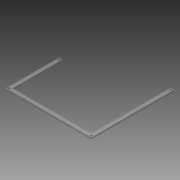
# Autodesk Inventor part: Bottom Plate
Saved by Autodesk Inventor 2013 (Build 170138000, 138)
## iProperties
Created: 2013-01-27
Part Number: Bottom Plate
Material: Polycarbonate, Clear
Document SubType Name: Modeling
Designer: Andrew Toennies
Density: 1.2 g/cm^3
Mass: 75.8926 g
Surface Area: 308.467 cm^2
Volume: 63.2438 cm^3
Author: Andrew Toennies
Autodesk Inventor part; units mm, degrees
ref_plane "YZ Plane" through (0, 0, 0) normal (1, 0, 0) x (0, 1, 0)
ref_plane "XZ Plane" through (0, 0, 0) normal (0, 1, 0) x (-1, 0, 0)
ref_plane "XY Plane" through (0, 0, 0) normal (0, 0, 1) x (1, 0, 0)
sketch "Sketch1" plane through (0, 0, 0) normal (0, 1, 0) x (-1, 0, 0)
  circle A0 centre (0, 0) radius 139.7
  line L0 (-146.05, 146.05) -> (-146.05, -146.05)
  line L1 (-146.05, -146.05) -> (0, -146.05)
  line L2 (-158.75, 158.75) -> (-158.75, -158.75)
  line L3 (-158.75, -158.75) -> (0, -158.75)
  line L4 (0, -158.75) -> (0, -146.05)
  line L5 (-146.05, 146.05) -> (146.05, 146.05)
  line L6 (146.05, 146.05) -> (146.05, -38.1)
  line L7 (146.05, -38.1) -> (158.75, -38.1)
  line L8 (158.75, -38.1) -> (158.75, 158.75)
  line L9 (158.75, 158.75) -> (-158.75, 158.75)
  dimension "d0" = 279.4
  dimension "d2" = 146.05
  dimension "d4" = 146.05
  dimension "d6" = 0
  dimension "d9" = 317.5
  dimension "d30" = 12.7
  dimension "d31" = 292.1
  dimension "d32" = 184.15
  dimension "d33" = 12.7
  dimension "d34" = 196.85
  constraints: 20 end point, 6 perpendicular, 3 parallel, 1 centre point, 1 coincident
  measures "d0" diameter of A0
  measures "d2" distance from line of L0 point (0, 0)
  measures "d4" distance of L1.end point (0, 0)
  measures "d6" horizontal distance of L1.end point (0, 0)
  measures "d9" distance of L2.start L2.end
  measures "d30" distance between parallel lines of L2 L0
  measures "d31" distance of L0.start L5.end
  measures "d32" distance of L5.end L6.end
  measures "d33" distance of L6.end L7.end
  measures "d34" distance of L7.end L8.end
extrude "Extrusion1" add sketch "Sketch1" along normal blind 6.35 contours L0 L1 L4 L3 L2 L9 L8 L7 L6 L5
sketch "Sketch2" plane through (0, 6.35, 0) normal (0, 1, 0) x (1, 0, 0)
  line L0 (-50.8, -158.75) -> (158.75, -158.75) projected
  line L1 (158.75, -158.75) -> (158.75, 158.75) projected
  line L2 (158.75, 158.75) -> (0, 158.75) projected
  line L3 (146.05, 146.05) -> (146.05, -146.05) projected
  line L4 (149.225, -149.225) -> (149.225, -155.575)
  line L5 (149.225, -155.575) -> (155.575, -155.575)
  line L6 (155.575, -155.575) -> (155.575, -149.225)
  line L7 (149.225, -149.225) -> (155.575, -149.225)
  line L8 (155.575, 146.05) -> (149.225, 146.05)
  line L9 (149.225, 146.05) -> (149.225, 139.7)
  line L10 (149.225, 139.7) -> (155.575, 139.7)
  line L11 (155.575, 139.7) -> (155.575, 146.05)
  point P0 (0, 0)
  dimension "d12" = 6.35
  dimension "d13" = 6.35
  dimension "d14" = 6.35
  dimension "d15" = 3.175
  dimension "d16" = 3.175
  dimension "d20" = 12.7
  dimension "d22" = 3.175
  dimension "d23" = 6.35
  dimension "d24" = 6.35
  constraints: 16 end point, 4 parallel, 2 perpendicular, 1 horizontal
  measures "d12" distance of L4.start L4.end
  measures "d13" distance of L4.end L5.end
  measures "d14" distance of L5.end L6.end
  measures "d15" distance between parallel lines of L0 L5
  measures "d16" distance between parallel lines of L1 L6
  measures "d20" distance between parallel lines of L2 L8
  measures "d22" distance between parallel lines of L1 L11
  measures "d23" distance of L8.start L8.end
  measures "d24" distance of L10.end L8.start
extrude "Extrusion2" cut sketch "Sketch2" against normal blind 6.35
sketch "Sketch3" plane through (0, 6.35, 0) normal (0, 1, 0) x (1, 0, 0)
  line L0 (158.75, -158.75) -> (158.75, 158.75) projected
  line L1 (158.75, 158.75) -> (0, 158.75) projected
  line L2 (0, 158.75) -> (0, 146.05) projected
  line L3 (0, 146.05) -> (146.05, 146.05) projected
  line L4 (146.05, 146.05) -> (146.05, -146.05) projected
  line L5 (146.05, 146.05) -> (146.05, 149.225)
  line L6 (146.05, 149.225) -> (158.75, 149.225)
  point P0 (0, 0)
  dimension "d27" = 3.175
  constraints: 4 end point, 1 collinear, 1 perpendicular, 1 point on line
  measures "d27" distance of L3.end L5.end
extrude "Extrusion3" cut sketch "Sketch3" against normal blind 25.4
sketch "Sketch4" plane through (0, 6.35, 0) normal (0, 1, 0) x (1, 0, 0)
  line L0 (-146.05, -146.05) -> (-146.05, 38.1) projected
  line L1 (-146.05, 38.1) -> (-158.75, 38.1) projected
  line L2 (-158.75, 38.1) -> (-158.75, -158.75) projected
  line L3 (-158.75, -158.75) -> (158.75, -158.75) projected
  line L4 (-155.575, -149.225) -> (-149.225, -149.225)
  line L5 (-149.225, -149.225) -> (-149.225, -155.575)
  line L6 (-149.225, -155.575) -> (-155.575, -155.575)
  line L7 (-155.575, -155.575) -> (-155.575, -149.225)
  line L8 (-155.575, 34.925) -> (-149.225, 34.925)
  line L9 (-149.225, 34.925) -> (-149.225, 28.575)
  line L10 (-149.225, 28.575) -> (-155.575, 28.575)
  line L11 (-155.575, 28.575) -> (-155.575, 34.925)
  point P0 (0, 0)
  dimension "d35" = 6.35
  dimension "d36" = 6.35
  dimension "d37" = 3.175
  dimension "d38" = 3.175
  dimension "d39" = 6.35
  dimension "d40" = 6.35
  dimension "d41" = 3.175
  dimension "d42" = 3.175
  constraints: 16 end point, 4 parallel, 2 horizontal, 2 perpendicular
  measures "d35" distance of L5.end L6.end
  measures "d36" distance of L4.end L5.end
  measures "d37" distance between parallel lines of L2 L7
  measures "d38" distance between parallel lines of L3 L6
  measures "d39" distance of L9.end L10.end
  measures "d40" distance of L8.end L9.end
  measures "d41" distance between parallel lines of L0 L9
  measures "d42" distance between parallel lines of L1 L8
extrude "Extrusion4" cut sketch "Sketch4" against normal blind 25.4
body "Solid1"
